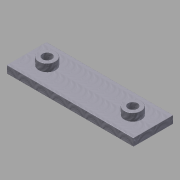
# Autodesk Inventor part: CIM MountBase
Saved by Autodesk Inventor 2013 (Build 170138000, 138)
## iProperties
Created: 2013-01-18
Part Number: CIM MountBase
Material: Aluminum 6061, Welded
Document SubType Name: Modeling
Designer: Naphat
Density: 1 g/cm^3
Author: Naphat
Autodesk Inventor part; units mm, degrees
ref_plane "YZ Plane" through (0, 0, 0) normal (1, 0, 0) x (0, 1, 0)
ref_plane "XZ Plane" through (0, 0, 0) normal (0, 1, 0) x (-1, 0, 0)
ref_plane "XY Plane" through (0, 0, 0) normal (0, 0, 1) x (1, 0, 0)
sketch "Sketch1" plane through (0, 0, 0) normal (0, 1, 0) x (-1, 0, 0)
  line L0 (0, 0) -> (284.48, 0)
  line L1 (284.48, 0) -> (284.48, 106.68)
  line L2 (284.48, 106.68) -> (0, 106.68)
  line L3 (0, 106.68) -> (0, 0)
  line L4 (0, 53.34) -> (27.305, 53.34) construction
  line L5 (284.48, 53.34) -> (257.175, 53.34) construction
  circle A0 centre (27.305, 53.34) radius 12.7
  circle A1 centre (257.175, 53.34) radius 12.7
  dimension "d0" = 284.48
  dimension "d1" = 106.68
  dimension "d2" = 27.305
  dimension "d3" = 27.305
  dimension "d4" = 25.4
  dimension "d5" = 25.4
  constraints: 12 end point, 3 perpendicular, 2 centre point, 2 coincident, 2 equal length, 2 midpoint, 1 horizontal
  measures "d0" distance of L0.start L0.end
  measures "d1" distance of L0.end L1.end
  measures "d2" distance of L4.start L4.end
  measures "d3" distance of L5.start L5.end
  measures "d4" diameter of A0
  measures "d5" diameter of A1
extrude "Extrusion1" add sketch "Sketch1" along normal blind 20.32
sketch "Sketch2" plane through (0, 20.32, 0) normal (0, 1, 0) x (1, 0, 0)
  circle A0 centre (-257.175, -53.34) radius 12.7 projected
  circle A1 centre (-27.305, -53.34) radius 12.7 projected
  circle A2 centre (-257.175, -53.34) radius 22.86
  circle A3 centre (-27.305, -53.34) radius 22.86
  dimension "d8" = 45.72
  dimension "d9" = 45.72
  constraints: 2 centre point, 2 coincident
  measures "d8" diameter of A2
  measures "d9" diameter of A3
extrude "Extrusion2" add sketch "Sketch2" along normal blind 20.32
sketch "Sketch3" plane through (-284.48, 0, 0) normal (-1, 0, 0) x (0, 0, 1)
  line L0 (0, 0) -> (106.68, 0) projected
  line L1 (106.68, 0) -> (106.68, 20.32) projected
  line L2 (0, 20.32) -> (106.68, 20.32) projected
  line L3 (0, 0) -> (0, 20.32) projected
extrude "Extrusion3" add sketch "Sketch3" along normal blind 27.94
sketch "Sketch4" plane through (0, 0, 106.68) normal (1, 0, 0) x (0, 0, -1)
  line L0 (0, 0) -> (106.68, 0) projected
  line L1 (106.68, 0) -> (106.68, 20.32) projected
  line L2 (0, 20.32) -> (106.68, 20.32) projected
  line L3 (0, 0) -> (0, 20.32) projected
extrude "Extrusion4" add sketch "Sketch4" along normal blind 27.94
fillet "Fillet1" radius 1 13 edges at (-312.42, 10.16, 106.68) (-142.24, 0, 106.68) (-142.24, 0, 0) (-312.42, 0, 53.34) (27.94, 0, 53.34) (27.94, 10.16, 106.68) (27.94, 10.16, 0) (-142.24, 20.32, 0) (27.94, 20.32, 53.34) (-142.24, 20.32, 106.68) (-312.42, 20.32, 53.34) (-280.035, 40.64, 53.34) (-50.165, 40.64, 53.34)
equation "\"d2\" = d3"
body "Solid1"
